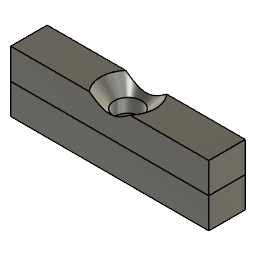
hexbug_3.5cm_mold_inprogress (Autodesk Fusion 360 design; units mm, degrees)
Autodesk Fusion 360 part; units mm, degrees
note: some values were not read from the file. Chosen so that the rebuilt part matches the saved one: which face or edge a step refers to. Set by a fixed rule: which sketch regions a step uses.
sketch "Sketch1" plane through (0, 0, 0) normal (0, 0, 1) x (1, 0, 0)
  line L0 (0, 0) -> (-65, 0)
  line L1 (-65, 0) -> (-65, 12)
  line L2 (-65, 12) -> (0, 12)
  line L3 (0, 12) -> (0, 0)
  dimension "d1" = 12
  dimension "d2" = 65
  constraint horizontal L0
  constraint vertical L1
  constraint horizontal L2
  constraint vertical L3
  constraint coincident L0.start L3.end
  measures "d1" distance of L0.start L2.end
  measures "d2" distance of L1.end L2.end
extrude "Extrude1" add sketch "Sketch1" along normal blind 10 makes body 1
sketch "Sketch2" plane through (0, 0, 10) normal (0, 0, 1) x (-1, 0, 0)
  line L0 (0, -12) -> (65, -12)
  line L1 (65, -12) -> (65, 0)
  line L2 (65, 0) -> (0, 0)
  line L3 (0, 0) -> (0, -12)
  line L4 (0, -6) -> (65, -6)
  line L5 (32.5, 0) -> (32.5, -12)
  line L6 (32.5, -6) -> (32.5, -8.5)
  line L7 (32.5, -6) -> (32.5, -3.5)
  line L8 (32.5, -8.5) -> (47.5, -8.5)
  line L9 (32.5, -3.5) -> (47.5, -3.5)
  line L10 (32.5, -3.5) -> (17.5, -3.5)
  line L11 (32.5, -8.5) -> (17.5, -8.5)
  circle A0 centre (17.5972, -6) radius 1
  circle A1 centre (47.5665, -6) radius 1
  circle A2 centre (17.5972, -6) radius 3.65
  circle A3 centre (47.5665, -6) radius 3.65
  dimension "d5" = 2.5
  dimension "d6" = 2.5
  dimension "d7" = 15
  dimension "d8" = 15
  dimension "d9" = 15
  dimension "d10" = 15
  dimension "d11" = 2
  dimension "d12" = 2
  dimension "d17" = 7.3
  dimension "d18" = 7.3
  constraint midpoint L3 L4.start
  constraint midpoint L1 L4.end
  constraint midpoint L2 L5.start
  constraint midpoint L0 L5.end
  constraint midpoint L4 L6.start
  constraint coincident L5 L6.end
  constraint perpendicular L4 L7
  constraint perpendicular L5 L8
  constraint perpendicular L5 L9
  constraint perpendicular L5 L10
  constraint perpendicular L6 L11
  measures "d5" distance of L6.start L6.end
  measures "d6" distance of L6.start L7.end
  measures "d7" distance of L6.end L8.end
  measures "d8" distance of L7.end L9.end
  measures "d9" distance of L7.end L10.end
  measures "d10" distance of L6.end L11.end
  measures "d11" diameter of A0
  measures "d12" diameter of A1
  measures "d17" diameter of A2
  measures "d18" diameter of A3
extrude "Extrude3" cut sketch "Sketch2" against normal blind 5 contours L4 L5 L6 L11 A2 | L4 L5 L6 L8 A3 | L4 L5 L7 L9 A3 | L4 L5 L7 L10 A2 | L4 A0 | L4 A0 | L4 A1 | L4 A1 bodies 1
extrude "Extrude4" cut sketch "Sketch2" against normal blind 5 contours L4 L5 L6 L11 A2 | L4 L5 L6 L8 A3 | L4 A0 A2 | L4 A0 A2 | L4 L5 L7 L9 A3 | L4 L5 L7 L10 A2 | L4 A1 A3 | L4 A1 A3 bodies 1
extrude "Extrude5" add sketch "Sketch2" against normal blind 5 contours L4 A0 | L4 A0 | L4 A1 | L4 A1 bodies 1
extrude "Extrude6" add sketch "Sketch2" along normal blind 10 bodies 1
sketch "Sketch3" plane through (0, 12, 0) normal (0, 1, 0) x (-1, 0, 0)
  line L0 (0, 0) -> (65, 0)
  line L1 (65, 0) -> (65, 20)
  line L2 (65, 20) -> (0, 20)
  line L3 (0, 20) -> (0, 0)
  line L4 (0, 20) -> (0, 10)
  line L5 (0, 10) -> (65, 10)
  constraint coincident L2.end L3.start
  constraint midpoint L3 L4.end
  constraint midpoint L1 L5.end
split "Split1" by curves path "Sketch3" along L4 L5 bodies 1 makes body 2 at (-43.3333, 4, 0)
sketch "Sketch4" plane through (0, 0, 10) normal (0, 0, 1) x (-1, 0, 0)
  arc A0 (20.2566, -3.5) -> (20.2566, -8.5) centre (17.5972, -6) ccw
  line L0 (20.2566, -3.5) -> (44.9071, -3.5)
  arc A1 (44.9071, -8.5) -> (44.9071, -3.5) centre (47.5665, -6) ccw
  line L1 (44.9071, -8.5) -> (20.2566, -8.5)
  line L2 (65, 0) -> (0, 0)
  line L3 (0, 0) -> (0, -12)
  line L4 (0, -12) -> (65, -12)
  line L5 (65, -12) -> (65, 0)
  line L6 (0, -6) -> (5, -6)
  circle A2 centre (5, -6) radius 1.25
  line L7 (65, -6) -> (60, -6)
  circle A3 centre (60, -6) radius 1.25
  dimension "d25" = 5
  dimension "d26" = 2.5
  dimension "d27" = 5
  dimension "d28" = 2.5
  constraint midpoint L3 L6.start
  constraint perpendicular L3 L6
  constraint coincident L6.end A2.centre
  constraint midpoint L5 L7.start
  constraint perpendicular L5 L7
  constraint coincident L7.end A3.centre
  measures "d25" distance of L6.start L6.end
  measures "d26" diameter of A2
  measures "d27" distance of L7.start L7.end
  measures "d28" diameter of A3
extrude "Extrude7" add sketch "Sketch4" along normal blind 2.5 contours A2 | A3 bodies 2
sketch "Sketch5" plane through (0, 0, 10) normal (0, 0, -1) x (1, 0, 0)
  line L0 (0, 0) -> (-65, 0)
  line L1 (-65, 0) -> (-65, -12)
  line L2 (-65, -12) -> (0, -12)
  line L3 (0, -12) -> (0, 0)
  line L4 (0, -6) -> (-5, -6)
  circle A0 centre (-5, -6) radius 1.25
  line L5 (-65, -6) -> (-60, -6)
  circle A1 centre (-60, -6) radius 1.25
  dimension "d31" = 5
  dimension "d32" = 2.5
  dimension "d33" = 5
  dimension "d34" = 2.5
  constraint midpoint L3 L4.start
  constraint perpendicular L3 L4
  constraint coincident L4.end A0.centre
  constraint midpoint L1 L5.start
  constraint perpendicular L1 L5
  constraint coincident L5.end A1.centre
  measures "d31" distance of L4.start L4.end
  measures "d32" diameter of A0
  measures "d33" distance of L5.start L5.end
  measures "d34" diameter of A1
extrude "Extrude8" cut sketch "Sketch5" against normal blind 2.5 contours A0 | A1 bodies 1
hole "Hole1" at (-32.5, 6, 20) direction (0, 0, -1) diameter 9 depth 9 tip angle 180 countersink diameter 18 countersink angle 90 bodies 1
extrude "Extrude2" cut sketch "Sketch2" against normal blind 2 contours L4 L5 L6 L11 A2 | L4 L5 L6 L8 A3 | L4 L5 L7 L9 A3 | L4 L5 L7 L10 A2 | L4 A0 | L4 A0 | L4 A1 | L4 A1 bodies 2
